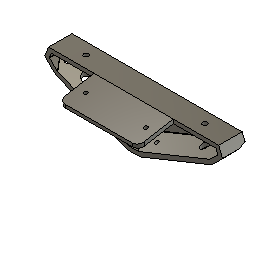
Psd2_Tof_bkt (Autodesk Fusion 360 design; units mm, degrees)
Autodesk Fusion 360 part; units mm, degrees
sketch "スケッチ1" plane through (0, 0, 0) normal (0, 0, 1) x (1, 0, 0)
  line L0 (-65, 0) -> (65, 0)
  line L1 (65, 0) -> (0, -26.2617)
  line L2 (0, -26.2617) -> (-65, 0)
  line L3 (46.0873, -7.6412) -> (43, 0)
  line L4 (-46.0873, -7.6412) -> (-43, 0)
  circle A0 centre (0, 35) radius 60
  dimension "d1" = 130
  dimension "d2" = 65
  dimension "d3" = 22
  dimension "d5" = 22
  dimension "d6" = 86
  dimension "d7" = 43
  dimension "d79" = 35
  dimension "d80" = 120
  constraint horizontal L0
  constraint coincident L1 L3.start
  constraint coincident L0 L3.end
  constraint perpendicular L1 L3
  constraint coincident L2 L4.start
  constraint coincident L0 L4.end
  constraint perpendicular L2 L4
  constraint coincident origin L0
  constraint vertical origin A0.centre
  measures "d1" distance of L0.start L0.end
  measures "d2" distance of origin L0.start
  measures "d3" angle of L0 L1
  measures "d5" angle of L0 L2
  measures "d6" distance of L3.end L4.end
  measures "d7" distance of origin L3.end
  measures "d79" distance of L0 A0.centre
  measures "d80" diameter of A0
extrude "押し出し1" add sketch "スケッチ1" along normal blind 12 contours L0 L1 L2 L3 L4 A0 | L2 L4 A0 | L1 L3 A0 | L1 L2 A0
sketch "スケッチ2" plane through (36.9658, 14.9352, 0) normal (0.927184, 0.374607, 0) x (0, 0, -1)
  line L0 (0, -24.3494) -> (0, -16.1081)
  line L1 (0, -16.1081) -> (-12, -16.1081)
  line L2 (-12, -16.1081) -> (-12, -24.3494)
  line L3 (-12, -24.3494) -> (0, -24.3494)
  line L4 (-12, -24.3494) -> (0, -19.9818)
  dimension "d10" = 20
  constraint coincident L2.end L3.start
  constraint coincident L0 L4.end
  measures "d10" angle of L3 L4
extrude "押し出し2" cut sketch "スケッチ2" against normal blind 93 contours L0 L3 L4
sketch "スケッチ3" plane through (-36.9658, 14.9352, 0) normal (-0.927184, 0.374607, 0) x (0, 0, 1)
  line L0 (0, -16.1081) -> (0, -24.3494)
  line L1 (0, -24.3494) -> (12, -24.3494)
  line L2 (12, -24.3494) -> (12, -16.1081)
  line L3 (12, -16.1081) -> (0, -16.1081)
  line L4 (12, -24.3494) -> (0, -19.9818)
  dimension "d13" = 20
  constraint coincident L1.end L2.start
  constraint coincident L0 L4.end
  measures "d13" angle of L1 L4
extrude "押し出し3" cut sketch "スケッチ3" against normal blind 70 contours L0 L1 L4
extrude "押し出し11" cut sketch "スケッチ1" along normal blind 20 contours L2 L4 A0 | L1 L3 A0 | L1 L2 A0
shell "シェル2" thickness 2 removed faces 1 at (0.373, -8.3299, 12)
sketch "スケッチ4" plane through (-6.6097, -16.3596, -6.422) normal (-0.352015, -0.871268, -0.34202) x (-0.696851, 0, 0.717216)
  line L0 (10.9447, -17.4132) -> (35.9237, 12.0943)
  line L1 (33.8097, 23.6151) -> (30.9758, 26.0141)
  circle A0 centre (32.0745, 16.8336) radius 1
  circle A1 centre (8.1684, -11.4064) radius 1
  line L2 (30.9758, 26.0141) -> (0, -10.5774)
  line L3 (0, -10.5774) -> (6.3014, -17.6045)
  ellipse E0 centre (-103.3214, 104.6429) end of major axis (-237.2161, 217.9888) minor radius 60 (35.9237, 12.0943) -> (33.8097, 23.6151) ccw
  ellipse E1 centre (-103.3214, 104.6429) end of major axis (-237.2161, 217.9888) minor radius 60 (6.3014, -17.6045) -> (10.9447, -17.4132) ccw
  dimension "d16" = 6
  dimension "d17" = 37
  dimension "d18" = 2
  dimension "d19" = 6
  dimension "d28" = 7
  constraint equal A0 A1
  measures "d16" distance of L0 A1.centre
  measures "d17" distance of A0.centre A1.centre
  measures "d18" diameter of A1
  measures "d19" distance of L0 A0.centre
  measures "d28" distance of L1.start A0.centre
extrude "押し出し4" cut sketch "スケッチ4" against normal blind 2 contours A0 | A1
sketch "スケッチ5" plane through (6.6097, -16.3596, -6.422) normal (0.352015, -0.871268, -0.34202) x (-0.696851, 0, -0.717216)
  line L0 (-30.9758, 26.0141) -> (-33.8097, 23.6151)
  line L1 (-35.9237, 12.0943) -> (-10.9447, -17.4132)
  circle A0 centre (-9.7678, -9.5172) radius 1
  circle A1 centre (-33.6738, 18.7229) radius 1
  line L2 (0, -10.5774) -> (-30.9758, 26.0141)
  line L3 (-6.3014, -17.6045) -> (0, -10.5774)
  ellipse E0 centre (103.3214, 104.6429) end of major axis (-30.5733, -8.7029) minor radius 60 (-33.8097, 23.6151) -> (-35.9237, 12.0943) ccw
  ellipse E1 centre (103.3214, 104.6429) end of major axis (-30.5733, -8.7029) minor radius 60 (-10.9447, -17.4132) -> (-6.3014, -17.6045) ccw
  dimension "d23" = 6
  dimension "d24" = 6
  dimension "d25" = 37
  dimension "d26" = 2
  dimension "d27" = 7
  constraint equal A0 A1
  measures "d23" distance of L1 A0.centre
  measures "d24" distance of L1 A1.centre
  measures "d25" distance of A0.centre A1.centre
  measures "d26" diameter of A0
  measures "d27" distance of L1.start A1.centre
extrude "押し出し5" cut sketch "スケッチ5" against normal blind 2 contours A0 | A1
sketch "スケッチ6" plane through (0, 0, 0) normal (0, 1, 0) x (-1, 0, 0)
  circle A0 centre (-30, 6) radius 1.2
  circle A1 centre (30, 6) radius 1.2
  line L0 (-30, 6) -> (30, 6)
  line L1 (30, 6) -> (-30, 6)
  line L2 (43, 12) -> (-43, 12)
  line L3 (-43, 12) -> (-43, 0)
  line L4 (-43, 0) -> (43, 0)
  line L5 (43, 0) -> (43, 12)
  circle A2 centre (-30, 6) radius 2
  circle A3 centre (30, 6) radius 2
  dimension "d36" = 60
  dimension "d37" = 30
  dimension "d39" = 2.4
  dimension "d50" = 6
  dimension "d91" = 4
  constraint coincident A0.centre L0.start
  constraint coincident A1.centre L0.end
  constraint equal A0 A1
  constraint horizontal L0
  constraint concentric A0 A2
  constraint concentric A1 A3
  constraint equal A2 A3
  measures "d36" distance of A0.centre A1.centre
  measures "d37" horizontal distance of origin A0.centre
  measures "d39" diameter of A1
  measures "d50" distance of L1 L2
  measures "d91" diameter of A2
extrude "押し出し6" cut sketch "スケッチ6" against normal blind 6 contours A0 | A1
extrude "押し出し12" cut sketch "スケッチ6" against normal blind 30 from surface at -2 contours A0 | A1 | A2 | A3
sketch "スケッチ7" plane through (0, 0, 2) normal (0, 0, 1) x (1, 0, 0)
  line L0 (46.1584, -8.6776) -> (43, 0)
  line L1 (43, 0) -> (-43, 0)
  line L2 (-43, 0) -> (-46.1584, -8.6776)
  line L3 (-46.1584, -8.6776) -> (0, -25.4779)
  line L4 (0, -25.4779) -> (46.1584, -8.6776)
  circle A0 centre (0, -9) radius 6
  line L5 (0, -23.0203) -> (-43.4892, -7.1915)
  line L6 (-43.4892, -7.1915) -> (-41.5996, -2)
  line L7 (-41.5996, -2) -> (41.5996, -2)
  line L8 (41.5996, -2) -> (43.4892, -7.1915)
  line L9 (43.4892, -7.1915) -> (0, -23.0203)
  line L10 (41.651, -2) -> (-41.651, -2)
  line L11 (-42.0721, -3.0424) -> (0, -20.0407)
  line L12 (0, -20.0407) -> (42.0721, -3.0424)
  line L13 (42.0721, -3.0424) -> (41.651, -2)
  line L14 (-41.651, -2) -> (-42.0721, -3.0424)
  dimension "d44" = 9
  dimension "d45" = 12
  constraint vertical origin A0.centre
  measures "d44" distance of origin A0.centre
  measures "d45" diameter of A0
extrude "押し出し8" cut sketch "スケッチ7" against normal blind 10 contours A0
sketch "スケッチ9" plane through (0, 0, 0) normal (1, 0, 0) x (0, 0, -1)
  line L0 (-12, 0) -> (-29.7265, -3.1257)
  line L1 (-29.7265, -3.1257) -> (-29.3792, -5.0953)
  line L2 (-29.3792, -5.0953) -> (-0.4825, 0)
  line L3 (0, 0) -> (-12, 0)
  line L4 (-12, 0) -> (-0.4825, 0)
  dimension "d70" = 18
  dimension "d71" = 2
  dimension "d72" = 10
  constraint perpendicular L0 L1
  constraint perpendicular L1 L2
  constraint coincident L0.start L3.end
  constraint coincident L2.end L3
  measures "d70" distance of L0.end L0.start
  measures "d71" distance of L0.end L2
  measures "d72" angle of L0 L3
extrude "押し出し10" add sketch "スケッチ9" along normal mid plane 40
sketch "スケッチ8" plane through (0, 2.0521, 0.3618) normal (0, 0.984808, 0.173648) x (-1, 0, 0)
  circle A0 centre (-30, 6) radius 0.9
  circle A1 centre (30, 6) radius 0.9
  line L0 (-43, 0) -> (43, 0)
  line L1 (43, 0) -> (43, 12)
  line L2 (-15, 12) -> (-43, 12)
  line L3 (-43, 12) -> (-43, 0)
  line L4 (-22.5, 12) -> (-22.5, 29)
  line L5 (-22.5, 29) -> (22.5, 29)
  line L6 (22.5, 29) -> (22.5, 12)
  circle A2 centre (-18.5, 22) radius 0.9
  circle A3 centre (18.5, 22) radius 0.9
  circle A4 centre (-15.25, 21) radius 0.9
  circle A5 centre (15.25, 21) radius 0.9
  line L7 (43, 12) -> (15, 12)
  line L8 (15, 12) -> (-15, 12)
  line L9 (20, 29.8177) -> (-20, 29.8177)
  line L10 (-20, 29.8177) -> (-20, 11.8177)
  line L11 (-20, 11.8177) -> (20, 11.8177)
  line L12 (20, 11.8177) -> (20, 29.8177)
  dimension "d54" = 45
  dimension "d55" = 22.5
  dimension "d56" = 17
  dimension "d59" = 1.8
  dimension "d60" = 37
  dimension "d61" = 18.5
  dimension "d62" = 10
  dimension "d67" = 8
  dimension "d68" = 30.5
  dimension "d69" = 15.25
  constraint coincident L2 L4.start
  constraint perpendicular L2 L4
  constraint perpendicular L4 L5
  constraint coincident L2 L6.end
  constraint perpendicular L2 L6
  constraint horizontal A2.centre A3.centre
  constraint equal A2 A3
  constraint horizontal A4.centre A5.centre
  constraint equal A2 A4
  constraint equal A4 A5
  measures "d54" distance of L4.end L5.end
  measures "d55" horizontal distance of origin L6.end
  measures "d56" distance of L5.end L6.end
  measures "d59" diameter of A2
  measures "d60" distance of A2.centre A3.centre
  measures "d61" horizontal distance of origin A3.centre
  measures "d62" vertical distance of L6.end A3.centre
  measures "d67" distance of L5 A5.centre
  measures "d68" distance of A4.centre A5.centre
  measures "d69" horizontal distance of origin A5.centre
extrude "押し出し9" cut sketch "スケッチ8" against normal blind 3 contours A4 | A5
fillet "フィレット7" radius 3 2 edges at (-20, -4.1105, 29.5529) (20, -4.1105, 29.5529)
fillet "フィレット9" radius 0.2 7 edges at (41.651, -2, 7) (42.3377, -3.6996, 3.9476) (0, -2, 2) (21.0361, -11.5415, 2) (-21.0361, -11.5415, 2) (-41.651, -2, 7) (-42.3377, -3.6996, 3.9476)
fillet "フィレット10" radius 0.2 3 edges at (-40.4907, -6.5271, 9.2494) (-42.581, -4.381, 6.2095) (-42.6032, -4.3569, 9.24)
fillet "フィレット11" radius 0.2 2 edges at (0, -21.5462, 5.8351) (0, -20.0133, 2.0362)
fillet "フィレット12" radius 0.2 1 faces at (-16.4695, -12.5075, 0)
equation "d2 = d1 / 2"
equation "d5 = d3"
equation "d7 = d6 / 2"
equation "d37 = d36 / 2"
equation "d55 = d54 / 2"
equation "d61 = d60 / 2"
equation "d69 = d68 / 2"
